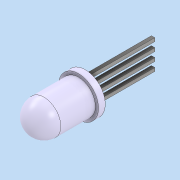
# Autodesk Inventor part: led
Saved by Autodesk Inventor 2020 (Build 240168000, 168)
## iProperties
Created: 2020-05-04
Part Number: led
Material: 일반
Document SubType Name: Modeling
Designer: sbahn
Density: 1 g/cm^3
Appearance: 기본값
Author: sbahn
Autodesk Inventor part; units mm, degrees
ref_plane "YZ Plane" through (0, 0, 0) normal (1, 0, 0) x (0, 1, 0)
ref_plane "XZ Plane" through (0, 0, 0) normal (0, 1, 0) x (-1, 0, 0)
ref_plane "XY Plane" through (0, 0, 0) normal (0, 0, 1) x (1, 0, 0)
sketch "스케치1" plane through (0, 0, 0) normal (1, 0, 0) x (0, 1, 0)
  line L0 (0, 0) -> (0, -8.6)
  line L1 (0, -8.6) -> (0, -25.7335)
  arc A0 (2.5, -2.5) -> (0, 0) centre (0, -2.5) ccw
  line L2 (2.5, -2.5) -> (2.5, -7.6)
  line L3 (0, -8.6) -> (2.95, -8.6)
  line L4 (2.95, -8.6) -> (2.95, -7.6)
  line L5 (2.95, -7.6) -> (2.5, -7.6)
  dimension "d0" = 8.6
  dimension "d1" = 17.1335
  dimension "d2" = 5
  dimension "d3" = 1
  dimension "d4" = 2.5
  dimension "d6" = 5.9
  constraints: 12 end point, 3 vertical, 2 perpendicular, 2 point on circle, 1 centre point, 1 horizontal, 1 point on line
  measures "d0" distance of L0.start L0.end
  measures "d1" distance of L0.end L1.end
  measures "d2" diameter of A0
  measures "d3" distance of L3.end L4.end
  measures "d4" distance between parallel lines of L0 L2
  measures "d6" diameter of L4 L1
revolve "회전1" add sketch "스케치1" angle 360 about axis through (0, 0, -8.6) along (0, 0, -1)
sketch "스케치2" plane through (0, 0, -8.6) normal (0, 0, -1) x (-1, 0, 0)
  line L0 (0.25, -1.655) -> (-0.25, -1.655)
  line L1 (-0.25, -1.655) -> (-0.25, -2.155)
  line L2 (-0.25, -2.155) -> (0.25, -2.155)
  line L3 (0.25, -2.155) -> (0.25, -1.655)
  line L4 (0.25, -1.655) -> (-0.25, -2.155) construction
  line L5 (-0.25, -1.655) -> (0.25, -2.155) construction
  line L6 (0.25, -0.385) -> (-0.25, -0.385)
  line L7 (-0.25, -0.385) -> (-0.25, -0.885)
  line L8 (-0.25, -0.885) -> (0.25, -0.885)
  line L9 (0.25, -0.885) -> (0.25, -0.385)
  line L10 (0.25, -0.385) -> (-0.25, -0.885) construction
  line L11 (-0.25, -0.385) -> (0.25, -0.885) construction
  line L12 (0.25, 0.885) -> (-0.25, 0.885)
  line L13 (-0.25, 0.885) -> (-0.25, 0.385)
  line L14 (-0.25, 0.385) -> (0.25, 0.385)
  line L15 (0.25, 0.385) -> (0.25, 0.885)
  line L16 (0.25, 0.885) -> (-0.25, 0.385) construction
  line L17 (-0.25, 0.885) -> (0.25, 0.385) construction
  line L18 (0.25, 2.155) -> (-0.25, 2.155)
  line L19 (-0.25, 2.155) -> (-0.25, 1.655)
  line L20 (-0.25, 1.655) -> (0.25, 1.655)
  line L21 (0.25, 1.655) -> (0.25, 2.155)
  line L22 (0.25, 2.155) -> (-0.25, 1.655) construction
  line L23 (-0.25, 2.155) -> (0.25, 1.655) construction
  line L24 (0, -1.905) -> (0, 1.905) construction
  point P0 (0, 0)
  point P1 (0, -0.635)
  point P2 (0, 0.635)
  point P3 (0, 0)
  point P4 (0, 0)
  dimension "d8" = 0.5
  dimension "d9" = 0.5
  dimension "d10" = 0.5
  dimension "d11" = 0.5
  dimension "d12" = 0.5
  dimension "d13" = 0.5
  dimension "d14" = 0.5
  dimension "d15" = 0.5
  dimension "d16" = 1.27
  dimension "d17" = 1.27
  dimension "d18" = 1.27
  constraints: 50 end point, 9 midpoint, 8 parallel, 4 horizontal, 4 perpendicular, 1 coincident, 1 vertical
  measures "d8" distance of L2.end L1.end
  measures "d9" distance of L1.end L0.end
  measures "d10" distance of L8.end L7.end
  measures "d11" distance of L7.end L6.end
  measures "d12" distance of L14.end L13.end
  measures "d13" distance of L13.end L12.end
  measures "d14" distance of L20.end L19.end
  measures "d15" distance of L19.end L18.end
  measures "d16" distance of point (0, 0.635) L24.end
  measures "d17" distance of point (0, -0.635) point (0, 0.635)
  measures "d18" distance of L24.start point (0, -0.635)
extrude "돌출1" add sketch "스케치2" along normal blind 10
equation "\"d17\" = d16"
equation "\"d18\" = d17"
